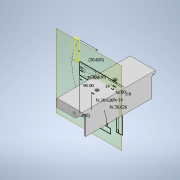
# Autodesk Inventor part: Capping_RotationAnchor
Saved by Autodesk Inventor 2022 (Build 260153000, 153)
## iProperties
Created: 2024-05-05
Part Number: Capping_RotationAnchor
Material: Generic
Document SubType Name: Modeling
Designer: raphael.hauk
Density: 1 g/cm^3
Appearance: Default
Author: raphael.hauk
Autodesk Inventor part; units mm, degrees
ref_plane "YZ Plane" through (0, 0, 0) normal (1, 0, 0) x (0, 1, 0)
ref_plane "XZ Plane" through (0, 0, 0) normal (0, 1, 0) x (-1, 0, 0)
ref_plane "XY Plane" through (0, 0, 0) normal (0, 0, 1) x (1, 0, 0)
ref_plane "Work Plane6" through (7.98, 0, 4.3086) normal (0, 0, 1) x (1, 0, 0)
sketch "Sketch1" plane through (0, 0, 0) normal (0, 0, 1) x (1, 0, 0)
  line L0 (7.98, 8) -> (7.98, -8) projected
  line L1 (7.98, 8) -> (3.98, 8) projected
  line L2 (3.98, -8) -> (3.98, 8) projected
  line L3 (7.98, -8) -> (3.98, -8) projected
  point P0 (0, 0)
  point P1 (21.25, -8.826)
  constraints: 2 other
sketch "Sketch2" plane through (0, 0, 0) normal (0, 0, 1) x (1, 0, 0)
  line L0 (17.98, -43.252) -> (33.98, -43.252)
  line L1 (33.98, -43.252) -> (33.98, -47.252)
  line L2 (33.98, -47.252) -> (17.98, -47.252)
  line L3 (17.98, -47.252) -> (17.98, -43.252)
  line L4 (3.98, -8) -> (3.98, 8) construction
  line L5 (7.98, 8) -> (3.98, 8) construction
  line L6 (7.98, 8) -> (7.98, -8) construction
  line L7 (7.98, -8) -> (3.98, -8) construction
  line L8 (38.606, -12.626) -> (7.98, -12.626) construction
  line L9 (38.606, -43.252) -> (38.606, -12.626) construction
  arc A0 (7.98, 8) -> (17.98, -43.252) centre (38.606, -12.626) ccw construction
  line L10 (21.25, -8.826) -> (0, -8.826) construction
  line L11 (7.98, -7.626) -> (38.606, -7.626)
  line L12 (38.606, -7.626) -> (38.606, -17.626)
  line L13 (38.606, -17.626) -> (7.98, -17.626)
  line L14 (7.98, -17.626) -> (7.98, -7.626)
  line L15 (7.98, -7.626) -> (38.606, -17.626) construction
  line L16 (38.606, -7.626) -> (7.98, -17.626) construction
  line L17 (38.606, -12.626) -> (38.606, -43.252)
  line L18 (38.606, -43.252) -> (43.606, -43.252)
  line L19 (43.606, -43.252) -> (43.606, -12.626)
  line L20 (43.606, -12.626) -> (38.606, -12.626)
  point P0 (38.606, -26.626)
  point P1 (24.606, -12.626)
  point P2 (23.293, -12.626)
  point P3 (7.98, 0)
  dimension "d3" = 20.626
  dimension "d5" = 20.626
  dimension "d6" = 30.626
  dimension "d7" = 30.626
  dimension "d8" = 3.8
  dimension "d9" = 30.626
  dimension "d26" = 14
  dimension "d27" = 14
  dimension "d44" = 10
  dimension "d47" = 5
  dimension "d82" = 10
  dimension "d83" = 90
  constraints: 34 end point, 8 equal length, 6 perpendicular, 5 midpoint, 5 point on line, 2 point on circle, 1 centre point, 1 coincident, 1 horizontal
  measures "d3" distance of L5.start L8.end
  measures "d5" distance of L0.start L9.start
  measures "d6" distance of L8.start L8.end
  measures "d7" distance of L9.start L8.start
  measures "d8" distance from line of L17.start L10
  measures "d9" distance from line of L6 L17.start
  measures "d26" distance of point (24.606, -12.626) L17.start
  measures "d27" distance of point (38.606, -26.626) L17.start
  measures "d44" distance of L11.end L12.end
  measures "d47" distance of L19.end L17.start
  measures "d82" horizontal distance of L0.start L6.end
  measures "d83" angle of L0 L6
ref_plane "Work Plane1" through (18.228, -8.826, 23.9001) normal (0, -1, 0) x (0, 0, -1)
sketch "Sketch3" plane through (18.228, -8.826, 23.9001) normal (0, -1, 0) x (0, 0, -1)
  circle A0 centre (11.5, 16.822) radius 1.45 construction
  circle A1 centre (26.5, 16.822) radius 1.45 construction
  circle A2 centre (11.5, 6.822) radius 1.45 construction
  circle A3 centre (26.5, 6.822) radius 1.45 construction
  line L0 (-12.9085, 5.822) -> (52.0915, 5.822)
  line L1 (52.0915, 5.822) -> (52.0915, 26.822)
  line L2 (52.0915, 26.822) -> (-12.9085, 26.822)
  line L3 (-12.9085, 26.822) -> (-12.9085, 5.822)
  line L4 (19.5915, -18.302) -> (19.5915, 38.076) construction
  point P0 (23.9001, -18.228)
  dimension "d10" = 10
  dimension "d11" = 1
  dimension "d55" = 65
  constraints: 10 end point, 2 parallel, 1 horizontal, 1 perpendicular, 1 vertical, 3 other
  measures "d10" distance from line of L2 A0.centre
  measures "d11" distance from line of L0 A2.centre
  measures "d55" distance of L1.end L2.end
extrude "Extrusion1" add sketch "Sketch3" along normal blind 2
ref_plane "Work Plane3" through (18.228, -12.826, 23.9001) normal (0, -1, 0) x (1, 0, 0)
sketch "Sketch4" plane through (18.228, -12.826, 23.9001) normal (0, -1, 0) x (1, 0, 0)
  point P0 (-18.228, -23.9001)
  point P1 (6.822, -11.5)
  point P2 (6.822, -26.5)
  point P3 (16.822, -11.5)
  point P4 (16.822, -26.5)
sketch "Sketch5" plane through (29.03, -8.826, 4.3086) normal (0, 0, 1) x (1, 0, 0)
  circle A0 centre (9.576, -3.8) radius 1.5
  line L0 (-4.98, -2) -> (16.02, -2) projected
  arc A1 (9.576, -6.8) -> (12.576, -3.8) centre (9.576, -3.8) ccw
  line L1 (9.576, -8.8) -> (-21.05, -8.8) construction
  line L2 (9.576, -8.8) -> (-5.424, -8.8) construction
  line L3 (-5.424, -8.8) -> (-5.424, -6.8) construction
  line L4 (-5.424, -6.8) -> (9.576, -6.8) construction
  line L5 (9.576, -6.8) -> (9.576, -8.8) construction
  line L6 (-5.424, -6.8) -> (9.576, -6.8)
  line L7 (14.576, -34.426) -> (14.576, -3.8) construction
  line L8 (14.576, -3.8) -> (14.576, -18.8) construction
  line L9 (14.576, -18.8) -> (12.576, -18.8) construction
  line L10 (12.576, -18.8) -> (12.576, -3.8) construction
  line L11 (12.576, -3.8) -> (14.576, -3.8)
  arc A2 (9.576, -6.8) -> (12.576, -3.8) centre (9.576, -3.8) ccw construction
  line L12 (14.576, -3.8) -> (16.02, -2)
  line L13 (-4.98, -2) -> (-4.98, -6.8)
  point P0 (-29.03, 8.826)
  point P1 (9.576, -3.8)
  point P2 (12.4103, -4.7834)
  point P3 (-4.7641, -2)
  dimension "d21" = 3
  dimension "d46" = 2
  dimension "d70" = 15
  constraints: 22 end point, 5 equal length, 5 point on line, 4 perpendicular, 4 point on circle, 3 centre point, 3 coincident, 1 tangent, 1 vertical
  measures "d21" diameter of A0
  measures "d46" distance between parallel lines of L1 L4
  measures "d70" distance of L9.end L10.end
extrude "Extrusion2" add sketch "Sketch5" along normal mid plane 65 contours A0 | L0 L12 L11 A1 L6 L13
ref_plane "Work Plane5" through (45.05, -8.826, 4.3086) normal (0, 0, -1) x (-1, 0, 0)
sketch "Sketch7" plane through (45.05, -8.826, 4.3086) normal (0, 0, -1) x (-1, 0, 0)
  line L0 (0, -2) -> (0, -18.8)
  line L1 (0, -18.8) -> (1.444, -18.8)
  line L2 (1.444, -3.8) -> (1.444, -18.8) construction
  line L3 (0, 0) -> (0, -2) construction
  line L4 (0, -2) -> (1.444, -3.8)
  line L5 (1.444, -18.8) -> (1.444, -3.8)
  line L6 (0, -2) -> (1.444, -3.8) projected
  line L7 (0, -2) -> (0, -6.4519)
  line L8 (0, -6.4519) -> (0, -18.8)
  point P0 (45.05, 8.826)
  point P1 (0, -2)
  constraints: 12 end point, 1 coincident, 1 collinear, 1 parallel, 1 perpendicular, 1 vertical
extrude "Extrusion3" add sketch "Sketch7" along normal mid plane 55
hole "Hole1" at (35.05, -12.826, 12.4001) at (35.05, -12.826, -2.5999) direction (0, 1, 0) diameter 2.6 end through all start extended yes counterbore diameter 5.5 counterbore depth 2 clearance for "Socket Head Cap Screw ISO 4762" size "M2.5" standard "ISO"
fillet "Fillet1" radius 1 2 edges at (44.328, -11.726, 31.8086) (44.328, -11.726, -23.1914)
sketch "Sketch8" plane through (38.606, -15.626, -28.1914) normal (0, -1, 0) x (1, 0, 0)
  circle A0 centre (-8.05, 50.5) radius 5.05
  line L0 (15.9809, 32.5) -> (-50.7776, 32.5) projected
  line L1 (0, 0) -> (0, 65) projected
  point P0 (-38.606, 28.1914)
  point P1 (0, 26.5631)
  point P2 (0, 39.6199)
  dimension "d56" = 10.1
  dimension "d57" = 8.05
  dimension "d84" = 18
  constraints: 1 centre point
  measures "d56" diameter of A0
  measures "d57" distance from line of A0.centre L1
  measures "d84" distance from line of L0 A0.centre
extrude "Extrusion4" cut sketch "Sketch8" against normal blind 1.2
sketch "Sketch9" plane through (43.606, -27.626, -23.1914) normal (-1, 0, 0) x (0, 0, 1)
  circle A0 centre (45.5, 7) radius 5.05
  line L0 (27.5, -30.6764) -> (27.5, 46.6764) projected
  line L1 (-5, 15) -> (-1, 15) projected
  line L2 (-1, 15) -> (56, 15) projected
  point P0 (23.1914, 27.626)
  point P1 (27.5, 15)
  point P2 (0, 15)
  dimension "d60" = 10.1
  dimension "d85" = 18
  dimension "d87" = 8
  constraints: 1 centre point
  measures "d60" diameter of A0
  measures "d85" distance from line of L0 A0.centre
  measures "d87" distance from line of A0.centre L2
extrude "Extrusion5" cut sketch "Sketch9" against normal blind 1.2
mirror "Mirror2" about plane through (45.05, -8.826, 4.3086) normal (0, 0, -1) of "Extrusion5", "Extrusion4"
sketch "Sketch10" plane through (24.05, -8.826, 36.8086) normal (0, 0, 1) x (1, 0, 0)
  point P0 (-24.05, 8.826)
  point P1 (14.556, -3.8)
hole "Hole2" at (38.606, -12.626, 36.8086) direction (0, 0, -1) diameter 2.1 depth 12 tip angle 118 clearance for "Socket Head Cap Screw ISO 4762" size "M2" standard "ISO"
ref_plane "Work Plane7" through (24.05, -8.826, 30.8086) normal (0, 0, 1) x (1, 0, 0)
sketch "Sketch11" plane through (24.05, -8.826, 30.8086) normal (0, 0, 1) x (1, 0, 0)
  circle A0 centre (14.556, -3.8) radius 1.05 projected
  line L0 (12.531, -2.6309) -> (14.556, -1.4617)
  line L1 (14.556, -1.4617) -> (16.581, -2.6309)
  line L2 (16.581, -2.6309) -> (16.581, -4.9691)
  line L3 (16.581, -4.9691) -> (14.556, -6.1383) construction
  line L4 (14.556, -6.1383) -> (12.531, -4.9691) construction
  line L5 (12.531, -4.9691) -> (12.531, -2.6309)
  line L6 (16.581, -4.9691) -> (16.581, -6.0135)
  arc A1 (14.556, -6.8) -> (17.556, -3.8) centre (14.556, -3.8) ccw projected
  line L7 (12.531, -4.9691) -> (12.531, -6.8)
  line L8 (0, -6.8) -> (14.556, -6.8) projected
  point P0 (-24.05, 8.826)
  point P1 (14.556, -3.8)
  point P2 (20.3903, -4.7834)
  point P3 (0.2159, -2)
  dimension "d79" = 4.05
  constraints: 16 end point, 3 vertical, 1 coincident, 1 point on circle, 15 other
  measures "d79" distance between parallel lines of L5 L2
extrude "Extrusion6" cut sketch "Sketch11" against normal blind 1.63 contours A0 | L0 L1 L2 L6 A1 L8 L7 L5
mirror "Mirror1" about plane through (45.05, -8.826, 4.3086) normal (0, 0, -1) of "Extrusion6", "Hole2"
sketch "Sketch12" plane through (24.05, -8.826, 36.8086) normal (0, 0, 1) x (1, 0, 0)
  line L0 (21, 0) -> (0, 0) projected
  line L1 (0, 0) -> (0, -6.8) projected
  line L2 (21, 0) -> (21, -2) projected
  line L3 (0, -6.8) -> (14.556, -6.8) projected
  arc A0 (14.556, -6.8) -> (17.556, -3.8) centre (14.556, -3.8) ccw projected
  line L4 (17.556, -3.8) -> (19.556, -3.8) projected
  line L5 (19.556, -3.8) -> (21, -2) projected
  point P0 (-24.05, 8.826)
extrude "Extrusion7" cut sketch "Sketch12" against normal blind 2
mirror "Mirror3" about plane through (45.05, -8.826, 4.3086) normal (0, 0, -1) of "Extrusion7"
equation "\"d5\" = d3"
equation "\"d7\" = d6"
equation "\"d27\" = d26"
equation "\"d47\" = 0.5 * d44"
body "Solid1"
